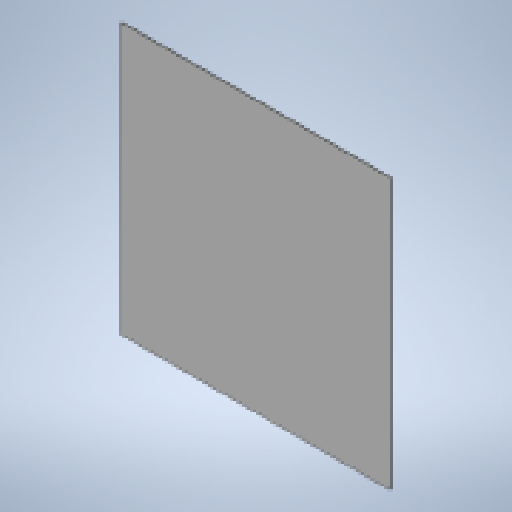
# Autodesk Inventor part: GBK 3339 shield 9
Saved by Autodesk Inventor 2026 (Build 300175000, 175)
## iProperties
Created: 2026-04-17
Part Number: GBK 3339 shield 9
Material: Steel
Document SubType Name: Sheet Metal
Designer: pokla
Stock Number: 3339
Mass: 69243.3 g
Surface Area: 44341.6 cm^2
Volume: 8820.8 cm^3
Density: 7.85 g/cm^3
Flat Pattern Width: 148 cm
Flat Pattern Length: 149 cm
Flat Pattern Area: 22052 cm^2
Sheet Metal Rule: По умолчанию_мм
Sheet Metal Width: 1480,000 мм
Sheet Metal Length: 1490,000 мм
Sheet Metal Area: 2205200,000 мм^2
Appearance: Default
Author: admin
Autodesk Inventor part; units mm, degrees
ref_plane "YZ Plane" through (0, 0, 0) normal (1, 0, 0) x (0, 1, 0)
ref_plane "XZ Plane" through (0, 0, 0) normal (0, 1, 0) x (-1, 0, 0)
ref_plane "XY Plane" through (0, 0, 0) normal (0, 0, 1) x (1, 0, 0)
sketch "Sketch1" plane through (0, 0, 0) normal (0, 0, 1) x (1, 0, 0)
  line L0 (740, -745) -> (-740, -745)
  line L1 (-740, -745) -> (-740, 745)
  line L2 (-740, 745) -> (740, 745)
  line L3 (740, 745) -> (740, -745)
  line L4 (740, -745) -> (-740, 745) construction
  line L5 (-740, -745) -> (740, 745) construction
  point P0 (0, 0)
  dimension "d0" = 1480
  dimension "d1" = 1490
  measures "d0" distance of L1.end L2.end
  measures "d1" distance of L0.end L1.end
extrude "Plate1" add sketch "Sketch1" along normal blind 4
sketch "Эскиз2" plane through (0, 0, 0) normal (0, 0, -1) x (-1, 0, 0)
  line L0 (582.7476, -597.0649) -> (582.7476, -1095.2011) construction
  line L1 (582.7476, -1095.2011) -> (543.1204, -1095.2011) construction
  line L2 (543.1204, -1095.2011) -> (543.1204, -597.0649) construction
  line L3 (543.1204, -597.0649) -> (582.7476, -597.0649) construction
  line L4 (209.363, -493) -> (209.363, -590) projected
  line L5 (209.363, -590) -> (205.363, -590) projected
  line L6 (-290.5101, -493) -> (-290.5101, -590) projected
  line L7 (-290.5101, -590) -> (-294.5101, -590) projected
  line L8 (-290.5101, 715) -> (-290.5101, 775) projected
  line L9 (-290.5101, 715) -> (-294.5101, 715) projected
  line L10 (209.363, 715) -> (209.363, 775) projected
  line L11 (209.363, 715) -> (205.363, 715) projected
  line L12 (739.6246, -489.5) -> (739.6246, -485.5) projected
  line L13 (739.6246, 7.1667) -> (739.6246, 11.1667) projected
  line L14 (739.6246, 503.8333) -> (739.6246, 507.8333) projected
  line L15 (-740, -489.5) -> (-710, -489.5) projected
  line L16 (-710, -489.5) -> (-710, -485.5) projected
  line L17 (-740, 7.1667) -> (-710, 7.1667) projected
  line L18 (-710, 7.1667) -> (-710, 11.1667) projected
  line L19 (-740, 503.8333) -> (-710, 503.8333) projected
  line L20 (-710, 503.8333) -> (-710, 507.8333) projected
  line L21 (739.6246, 503.8333) -> (709.6246, 503.8333)
  line L22 (739.6246, 7.1667) -> (709.6246, 7.1667)
  line L23 (739.6246, -489.5) -> (709.6246, -489.5)
  point P0 (0, 0)
  dimension "d6" = 30
  dimension "d7" = 30
  dimension "d8" = 30
  constraints: 6 end point, 3 horizontal, 2 other
  measures "d6" distance of L14.start L21.end
  measures "d7" distance of L22.start L22.end
  measures "d8" distance of L23.start L23.end
mark "Маркировка1"
equation "\"d0\" = Лист_ширина"
equation "\"d1\" = 0.5 * Лист_длина"
equation "\"d2\" = Thickness"
equation "\"BendRadius\" = Thickness"
equation "\"BendReliefWidth\" = Thickness"
equation "\"BendReliefDepth\" = 0.5 * Thickness"
equation "\"CornerReliefSize\" = 4 * Thickness"
equation "\"MinimumRemnant\" = 2 * Thickness"
equation "\"TransitionRadius\" = BendRadius"
equation "\"JacobiRadiusSize\" = BendRadius"
equation "\"GapSize\" = Thickness"
equation "\"Лист_ширина\" = 1480"
equation "\"Лист_длина\" = 2980"
equation "\"Thickness\" = 4"
body "Solid1"
